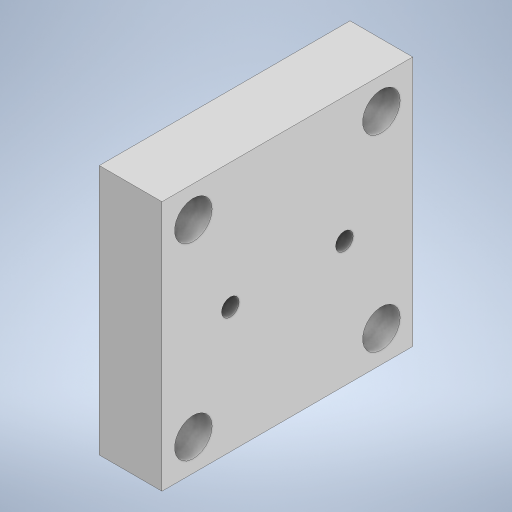
# Autodesk Inventor part: AdapterplatteGong_2025-03-27v00r00grm
Saved by Autodesk Inventor 2023 (Build 270158000, 158)
## iProperties
Created: 2025-03-27
Part Number: AdapterplatteGong_2025-03-27v00r00grm
Material: Generisch
Document SubType Name: Modeling
Designer: student
Density: 1 g/cm^3
Appearance: Vorgabe
Author: student
Autodesk Inventor part; units mm, degrees
ref_plane "YZ Plane" through (0, 0, 0) normal (1, 0, 0) x (0, 1, 0)
ref_plane "XZ Plane" through (0, 0, 0) normal (0, 1, 0) x (-1, 0, 0)
ref_plane "XY Plane" through (0, 0, 0) normal (0, 0, 1) x (1, 0, 0)
sketch "Skizze1" plane through (0, 0, 0) normal (1, 0, 0) x (0, 1, 0)
  line L0 (20, 20) -> (-20, 20)
  line L1 (-20, 20) -> (-20, -20)
  line L2 (-20, -20) -> (20, -20)
  line L3 (20, -20) -> (20, 20)
  point P0 (0, 0)
  dimension "d0" = 40
  dimension "d1" = 40
  dimension "d2" = 20
  dimension "d3" = 20
  constraints: 8 end point, 2 parallel, 1 horizontal, 1 perpendicular
  measures "d0" distance of L2.end L0.start
  measures "d1" distance of L1.end L2.end
  measures "d2" distance from line of point (0, 0) L3
  measures "d3" distance from line of point (0, 0) L2
extrude "Extrusion1" add sketch "Skizze1" along normal blind 10
sketch "Skizze2" plane through (10, 0, 0) normal (1, 0, 0) x (0, 0, -1)
  circle A0 centre (-15, 15) radius 3
  circle A1 centre (-15, -15) radius 3
  circle A2 centre (15, -15) radius 3
  circle A3 centre (15, 15) radius 3
  point P0 (0, 0)
  point P1 (0, 0)
  dimension "d7" = 6
  dimension "d8" = 15
  dimension "d9" = 15
  dimension "d14" = 360
  constraints: 4 centre point, 1 coincident, 9 other
  measures "d7" diameter of A0
  measures "d8" horizontal distance of point (0, 0) A0.centre
  measures "d9" horizontal distance of point (0, 0) A0.centre
extrude "Extrusion2" cut sketch "Skizze2" against normal through all
sketch "Skizze3" plane through (10, 0, 0) normal (1, 0, 0) x (0, 0, -1)
  circle A0 centre (-9.1, 0) radius 1.4
  line L0 (0, 22.3983) -> (0, -21.9034) construction
  circle A1 centre (9.1, 0) radius 1.4
  point P0 (0, 0)
  dimension "d16" = 2.8
  dimension "d17" = 9.1
  constraints: 2 centre point, 2 end point, 1 horizontal alignment, 1 point on line, 1 symmetric about line, 1 vertical, 1 other
  measures "d16" diameter of A0
  measures "d17" distance of A0.centre point (0, 0)
extrude "Extrusion3" cut sketch "Skizze3" against normal through all
